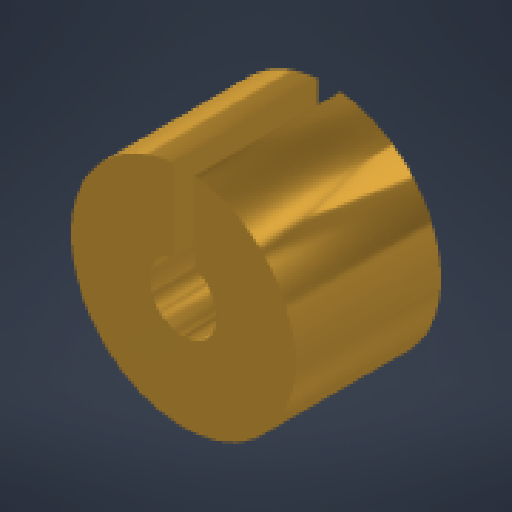
# Autodesk Inventor part: Reducer bushing
Saved by Autodesk Inventor 2026.3 (Build 303398000, 398)
## iProperties
Created: 2026-05-27
Part Number: Reducer bushing
Material: Generic
Document SubType Name: Sheet Metal
Designer: matot
Density: 1 g/cm^3
Sheet Metal Rule: Default_mm
Appearance: Default
Author: matot
Autodesk Inventor part; units mm, degrees
ref_plane "YZ Plane" through (0, 0, 0) normal (1, 0, 0) x (0, 1, 0)
ref_plane "XZ Plane" through (0, 0, 0) normal (0, 1, 0) x (-1, 0, 0)
ref_plane "XY Plane" through (0, 0, 0) normal (0, 0, 1) x (1, 0, 0)
sketch "Sketch1" plane through (0, 0, 0) normal (0, 0, 1) x (1, 0, 0)
  arc A0 (-1.6583, 2.5) -> (1.6583, 2.5) centre (0, 0) ccw
  arc A1 (-1, 9.9499) -> (1.0526, 9.9444) centre (0, 0) ccw
  line L0 (1.0526, 2.5) -> (1.0526, 9.9444)
  line L1 (-1, 9.9499) -> (-1, 2.5)
  line L2 (-1.6583, 2.5) -> (-1, 2.5)
  line L3 (1.0526, 2.5) -> (1.6583, 2.5)
  dimension "d0" = 6
  dimension "d2" = 20
  dimension "d4" = 1
  constraints: 8 end point, 4 point on circle, 2 centre point, 2 coincident, 2 horizontal, 1 parallel
  measures "d0" diameter of A0
  measures "d2" diameter of A1
  measures "d4" distance from line of point (0, 0) L1
extrude "Extrusion1" add sketch "Sketch1" along normal blind 13
equation "\"BendRadius\" = Thickness"
equation "\"BendReliefWidth\" = Thickness"
equation "\"BendReliefDepth\" = 0.5 * Thickness"
equation "\"CornerReliefSize\" = 4 * Thickness"
equation "\"MinimumRemnant\" = 2 * Thickness"
equation "\"TransitionRadius\" = BendRadius"
equation "\"JacobiRadiusSize\" = BendRadius"
equation "\"GapSize\" = Thickness"
equation "\"Thickness\" = 0.5"
body "Solid1"
